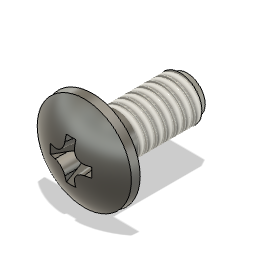
left handed writing device v4 (Autodesk Fusion 360 archive; units mm, degrees)
design "Type I Cross Recessed Binding Head Machine Screw ANSI B18.6.3 0-80 UNF x 0.125 Steel Grade 2 Plain"
description: Type I Cross Recessed Binding Head Machine Screw ANSI B18.6.3 0-80 UNF x 0.125
Autodesk Fusion 360 part; units mm, degrees
sketch "Sketch1" plane through (0, 0, 0) normal (0, 1, 0) x (1, 0, 0)
  line L0 (-0.762, 0) -> (-0.762, 3.175)
  line L1 (-0.762, 3.175) -> (0, 3.175)
  line L2 (0, 3.175) -> (0, -0.8128)
  line L3 (-0.762, 0) -> (-1.6002, 0)
  line L4 (-1.6002, 0) -> (-1.5766, -0.2698)
  arc A0 (-1.5766, -0.2698) -> (0, -0.8128) centre (0, 1.7475) ccw
  dimension "d9" = 1.524
  dimension "d66" = 3.2004
  dimension "d67" = 0.8128
  dimension "d68" = 3.175
  dimension "d70" = 2.5603
  dimension "d86" = 85
  constraint perpendicular L0 L1
  constraint collinear origin L2.end L1.end
  constraint perpendicular L0 L3
  constraint coincident origin L3
  constraint vertical L0
  constraint vertical L2
  constraint coincident L2 A0.centre
  measures "d67" vertical distance of L2.end L3.end
  measures "d68" distance of origin L1.end
  measures "d70" radius of A0
  measures "d86" angle of L3 L4
revolve "Revolve1" add sketch "Sketch1" angle 360 about axis through (0, 0, -3.175) along (0, 0, 1) makes body 1
ref_plane "WorkPlane1" through (0, 0, 0.8128) normal (0, 0, 1) x (1, 0, 0)
sketch "Sketch2" plane through (0, 0, 0.8128) normal (0, 0, 1) x (1, 0, 0)
  circle A0 centre (0, 0) radius 3
  line L0 (-0.1651, 0.762) -> (-0.1651, 0.1651)
  line L1 (-0.1651, 0.1651) -> (-0.762, 0.1651)
  line L2 (0, 0) -> (0, 0.762) construction
  line L3 (0.1651, 0.1651) -> (0.762, 0.1651)
  line L4 (0.1651, 0.762) -> (0.1651, 0.1651)
  line L5 (0.1651, -0.1651) -> (0.762, -0.1651)
  line L6 (0.1651, -0.762) -> (0.1651, -0.1651)
  line L7 (-0.1651, -0.762) -> (-0.1651, -0.1651)
  line L8 (-0.1651, -0.1651) -> (-0.762, -0.1651)
  line L9 (-0.1651, 0.762) -> (0.1651, 0.762)
  line L10 (-0.762, 0.1651) -> (-0.762, -0.1651)
  line L11 (-0.1651, -0.762) -> (0.1651, -0.762)
  line L12 (0.762, -0.1651) -> (0.762, 0.1651)
  line L13 (1.75, 0) -> (22.5, 0)
  circle A1 centre (0, 0) radius 1.5
  dimension "d22" = 0.3302
  dimension "d57" = 1.524
  constraint perpendicular L0 L1
  constraint coincident A0.centre L2.start
  constraint symmetric L0.start L2 L4.start
  constraint symmetric L0.end L2 L3.start
  constraint symmetric L1.end L2 L3.end
  constraint perpendicular L4 L9
  constraint perpendicular L8 L10
  constraint equal L9 L10
  constraint equal L0 L1
  constraint symmetric L1 L8 L13
  constraint horizontal L0.start L2.end
  constraint vertical L2
  constraint symmetric L3 L5 L13
  constraint symmetric L2 L6 L7
  constraint symmetric L9 L11 L13
  constraint collinear L4 L6
  measures "d22" horizontal distance of L0.start L4.start
  measures "d57" distance of L10 L12
extrude "Extrude1" add sketch "Sketch2" against normal blind 0.7874 draft -4 separate body contours L0 L1 L3 L4 L5 L6 L7 L8 L9 L10 L11 L12 makes body 2
draft "Draft1" angle -30 neutral plane through (0, 0, 0.8128) pull (0, 0, 1) 4 faces at (0.7436, 0.0367, 0.5503) (-0.0367, 0.7436, 0.5503) (-0.7436, 0.0367, 0.5503) (0.0367, -0.7436, 0.5503) on bodies 2
fillet "Fillet3" radius 0.3302 4 edges at (-0.1376, 0.1376, 0.4191) (0.1376, 0.1376, 0.4191) (0.1376, -0.1376, 0.4191) (-0.1376, -0.1376, 0.4191) on bodies 2
combine "Combine1" operation cut target body 1 tool bodies 2
thread "Thread2" "ANSI Unified Screw Threads 0.06(#0) 0-80 UNF 2A" major diameter 1.4707 minor diameter 1.1328 pitch 0.3175 angle 60 resizes the face on face at (-0.7582, 0.0759, -1.0583) from (0, 0, -0.7937) to (0, 0, -3.175) on bodies 1
sketch "Sketch5" plane through (0, 0, 0) normal (0, 1, 0) x (1, 0, 0)
  line L0 (0, -1.75) -> (0, -22.5)
  line L1 (0, 3.175) -> (0, -0.8128)
  line L2 (0, 3.175) -> (-0.7772, 3.175)
  line L3 (-0.7772, 3.175) -> (-0.7772, 2.8575)
  line L4 (-0.7772, 2.8575) -> (-0.6032, 3.175)
  dimension "d98" = 0.6033
  dimension "d99" = 0.7772
  dimension "d100" = 0.3175
  constraint coincident L1.start L2.start
  constraint perpendicular L1 L2
  constraint perpendicular L2 L3
  constraint coincident L2 L4.end
  measures "d98" horizontal distance of origin L4.end
  measures "d99" horizontal distance of origin L2.end
  measures "d100" distance of L2.end L3.end
revolve "Revolve2" cut sketch "Sketch5" angle 360 about axis through (0, 0, -3.175) along (0, 0, 1) bodies 1
equation "d9 = adsk_nomdia"
equation "d22 = adsk_philwidth"
equation "d31 = -adsk_phildepth"
equation "d57 = adsk_phildia"
equation "d59 = adsk_philwidth"
equation "d66 = adsk_headdia"
equation "d67 = adsk_headh"
equation "d68 = adsk_nomlen"
equation "d70 = adsk_headdia * 0.8"
equation "d71 = adsk_headh"
equation "adsk_nomlen = 0.125 in"
equation "adsk_headh = 0.032 in"
equation "adsk_headdia = 0.126 in"
equation "adsk_nomdia = 0.06 in"
equation "adsk_phildia = 0.06 in"
equation "adsk_philwidth = 0.013 in"
equation "adsk_phildepth = 0.031 in"
equation "adsk_thrlen = 0.09375 in"
equation "d84 = adsk_thrlen"
equation "adsk_startlen = 0.0125 in"
equation "adsk_endpointdia = 0.0475 in"
equation "d98 = adsk_endpointdia / 2"
equation "d99 = adsk_nomdia * 0.51"
equation "d100 = adsk_startlen"
